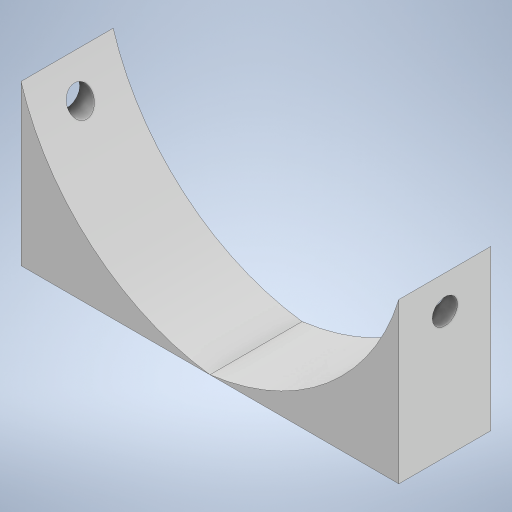
# Autodesk Inventor part: stand111
Saved by Autodesk Inventor 2023 (Build 270158000, 158)
## iProperties
Created: 2025-04-16
Part Number: stand111
Material: Generic
Document SubType Name: Modeling
Designer: dhara
Density: 1 g/cm^3
Appearance: Default
Author: dhara
Autodesk Inventor part; units mm, degrees
ref_plane "YZ Plane" through (0, 0, 0) normal (1, 0, 0) x (0, 1, 0)
ref_plane "XZ Plane" through (0, 0, 0) normal (0, 1, 0) x (-1, 0, 0)
ref_plane "XY Plane" through (0, 0, 0) normal (0, 0, 1) x (1, 0, 0)
sketch "Sketch1" plane through (0, 0, 0) normal (0, 0, 1) x (1, 0, 0)
  line L0 (2082.8, 9.2367) -> (2082.8, -879.7633)
  line L1 (2082.8, -879.7633) -> (1041.4, -879.7633)
  line L2 (1041.4, -879.7633) -> (1041.4, 9.2367) construction
  arc A0 (1041.4, -879.7633) -> (2082.8, 0) centre (878.782, 368.9807) ccw
  line L3 (0, 9.2367) -> (0, -879.7633)
  line L4 (0, -879.7633) -> (1041.4, -879.7633)
  arc A1 (0, 0) -> (1041.4, -879.7633) centre (1204.018, 368.9807) ccw
  point P0 (0, 0)
  constraints: 10 end point, 4 point on circle, 4 symmetric about line, 2 centre point, 2 point on line, 1 parallel, 1 other
extrude "Extrusion1" add sketch "Sketch1" along normal mid plane 508
sketch "Sketch2" plane through (2082.8, -879.7633, 254) normal (1, 0, 0) x (0, 0, -1)
  circle A0 centre (254, 696.6326) radius 69.7954
  point P0 (254, 879.7633)
  constraints: 1 centre point
extrude "Extrusion2" cut sketch "Sketch2" against normal blind 2381.25
body "Solid1"
